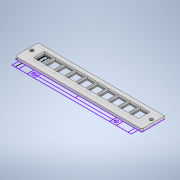
# Autodesk Inventor part: led strip face plate w label addon
Saved by Autodesk Inventor 2022 (Build 260153000, 153)
## iProperties
Created: 2022-04-12
Part Number: led strip face plate w label addon
Material: Generic
Document SubType Name: Modeling
Designer: a-dubs
Density: 1 g/cm^3
Appearance: Default
Author: a-dubs
Autodesk Inventor part; units mm, degrees
ref_plane "YZ Plane" through (0, 0, 0) normal (1, 0, 0) x (0, 1, 0)
ref_plane "XZ Plane" through (0, 0, 0) normal (0, 1, 0) x (-1, 0, 0)
ref_plane "XY Plane" through (0, 0, 0) normal (0, 0, 1) x (1, 0, 0)
sketch "Sketch1" plane through (0, 0, 0) normal (0, 1, 0) x (-1, 0, 0)
  line L0 (0, 0) -> (-9.9, 0)
  line L1 (0, 0) -> (0, -10.3)
  line L2 (0, -10.3) -> (-9.9, -10.3)
  line L3 (-9.9, -10.3) -> (-9.9, 0)
  line L4 (-9.9, -10.3) -> (-9.4, -10.3)
  line L5 (-9.4, -10.3) -> (-9.4, 0)
  line L6 (0, -10.3) -> (-0.5, -10.3)
  line L7 (-0.5, -10.3) -> (-0.5, 0)
  line L8 (-0.5, 0.85) -> (-9.9, 0.85)
  line L9 (-9.9, 0.85) -> (-9.9, 0)
  line L10 (0, 0) -> (0, 0.85)
  line L11 (0, 0.85) -> (-0.5, 0.85)
  line L12 (0, -10.3) -> (0, -11.15)
  line L13 (0, -11.15) -> (-9.9, -11.15)
  line L14 (-9.9, -11.15) -> (-9.9, -10.3)
  line L15 (-9.9, -11.15) -> (-19.8, -11.15)
  line L16 (-19.8, -11.15) -> (-19.8, -10.3)
  line L17 (-19.8, -10.3) -> (-19.8, 0)
  line L18 (-19.3, -10.3) -> (-19.3, 0)
  line L19 (-9.9, -10.3) -> (-19.8, -10.3)
  line L20 (-10.4, -10.3) -> (-10.4, 0)
  line L21 (-9.9, 0) -> (-9.9, -10.3)
  line L22 (-9.9, 0) -> (-9.9, 0.85)
  line L23 (-9.9, 0.85) -> (-10.4, 0.85)
  line L24 (-10.4, 0.85) -> (-19.8, 0.85)
  line L25 (-9.9, 0) -> (-19.8, 0)
  line L26 (-19.8, 0.85) -> (-19.8, 0)
  line L27 (-19.8, -11.15) -> (-29.7, -11.15)
  line L28 (-29.7, -11.15) -> (-29.7, -10.3)
  line L29 (-29.7, -10.3) -> (-29.7, 0)
  line L30 (-29.2, -10.3) -> (-29.2, 0)
  line L31 (-19.8, -10.3) -> (-29.7, -10.3)
  line L32 (-20.3, -10.3) -> (-20.3, 0)
  line L33 (-19.8, 0) -> (-19.8, -10.3)
  line L34 (-19.8, 0) -> (-19.8, 0.85)
  line L35 (-19.8, 0.85) -> (-20.3, 0.85)
  line L36 (-20.3, 0.85) -> (-29.7, 0.85)
  line L37 (-19.8, 0) -> (-29.7, 0)
  line L38 (-29.7, 0.85) -> (-29.7, 0)
  line L39 (-29.7, -11.15) -> (-39.6, -11.15)
  line L40 (-39.6, -11.15) -> (-39.6, -10.3)
  line L41 (-39.6, -10.3) -> (-39.6, 0)
  line L42 (-39.1, -10.3) -> (-39.1, 0)
  line L43 (-29.7, -10.3) -> (-39.6, -10.3)
  line L44 (-30.2, -10.3) -> (-30.2, 0)
  line L45 (-29.7, 0) -> (-29.7, -10.3)
  line L46 (-29.7, 0) -> (-29.7, 0.85)
  line L47 (-29.7, 0.85) -> (-30.2, 0.85)
  line L48 (-30.2, 0.85) -> (-39.6, 0.85)
  line L49 (-29.7, 0) -> (-39.6, 0)
  line L50 (-39.6, 0.85) -> (-39.6, 0)
  line L51 (-39.6, -11.15) -> (-49.5, -11.15)
  line L52 (-49.5, -11.15) -> (-49.5, -10.3)
  line L53 (-49.5, -10.3) -> (-49.5, 0)
  line L54 (-49, -10.3) -> (-49, 0)
  line L55 (-39.6, -10.3) -> (-49.5, -10.3)
  line L56 (-40.1, -10.3) -> (-40.1, 0)
  line L57 (-39.6, 0) -> (-39.6, -10.3)
  line L58 (-39.6, 0) -> (-39.6, 0.85)
  line L59 (-39.6, 0.85) -> (-40.1, 0.85)
  line L60 (-40.1, 0.85) -> (-49.5, 0.85)
  line L61 (-39.6, 0) -> (-49.5, 0)
  line L62 (-49.5, 0.85) -> (-49.5, 0)
  line L63 (-49.5, -11.15) -> (-59.4, -11.15)
  line L64 (-59.4, -11.15) -> (-59.4, -10.3)
  line L65 (-59.4, -10.3) -> (-59.4, 0)
  line L66 (-58.9, -10.3) -> (-58.9, 0)
  line L67 (-49.5, -10.3) -> (-59.4, -10.3)
  line L68 (-50, -10.3) -> (-50, 0)
  line L69 (-49.5, 0) -> (-49.5, -10.3)
  line L70 (-49.5, 0) -> (-49.5, 0.85)
  line L71 (-49.5, 0.85) -> (-50, 0.85)
  line L72 (-50, 0.85) -> (-59.4, 0.85)
  line L73 (-49.5, 0) -> (-59.4, 0)
  line L74 (-59.4, 0.85) -> (-59.4, 0)
  line L75 (-59.4, -11.15) -> (-69.3, -11.15)
  line L76 (-69.3, -11.15) -> (-69.3, -10.3)
  line L77 (-69.3, -10.3) -> (-69.3, 0)
  line L78 (-68.8, -10.3) -> (-68.8, 0)
  line L79 (-59.4, -10.3) -> (-69.3, -10.3)
  line L80 (-59.9, -10.3) -> (-59.9, 0)
  line L81 (-59.4, 0) -> (-59.4, -10.3)
  line L82 (-59.4, 0) -> (-59.4, 0.85)
  line L83 (-59.4, 0.85) -> (-59.9, 0.85)
  line L84 (-59.9, 0.85) -> (-69.3, 0.85)
  line L85 (-59.4, 0) -> (-69.3, 0)
  line L86 (-69.3, 0.85) -> (-69.3, 0)
  line L87 (-69.3, -11.15) -> (-79.2, -11.15)
  line L88 (-79.2, -11.15) -> (-79.2, -10.3)
  line L89 (-79.2, -10.3) -> (-79.2, 0)
  line L90 (-78.7, -10.3) -> (-78.7, 0)
  line L91 (-69.3, -10.3) -> (-79.2, -10.3)
  line L92 (-69.8, -10.3) -> (-69.8, 0)
  line L93 (-69.3, 0) -> (-69.3, -10.3)
  line L94 (-69.3, 0) -> (-69.3, 0.85)
  line L95 (-69.3, 0.85) -> (-69.8, 0.85)
  line L96 (-69.8, 0.85) -> (-79.2, 0.85)
  line L97 (-69.3, 0) -> (-79.2, 0)
  line L98 (-79.2, 0.85) -> (-79.2, 0)
  line L99 (-79.2, -11.15) -> (-89.1, -11.15)
  line L100 (-89.1, -11.15) -> (-89.1, -10.3)
  line L101 (-89.1, -10.3) -> (-89.1, 0)
  line L102 (-88.6, -10.3) -> (-88.6, 0)
  line L103 (-79.2, -10.3) -> (-89.1, -10.3)
  line L104 (-79.7, -10.3) -> (-79.7, 0)
  line L105 (-79.2, 0) -> (-79.2, -10.3)
  line L106 (-79.2, 0) -> (-79.2, 0.85)
  line L107 (-79.2, 0.85) -> (-79.7, 0.85)
  line L108 (-79.7, 0.85) -> (-89.1, 0.85)
  line L109 (-79.2, 0) -> (-89.1, 0)
  line L110 (-89.1, 0.85) -> (-89.1, 0)
  line L111 (-89.1, -11.15) -> (-99, -11.15)
  line L112 (-99, -11.15) -> (-99, -10.3)
  line L113 (-99, -10.3) -> (-99, 0)
  line L114 (-98.5, -10.3) -> (-98.5, 0)
  line L115 (-89.1, -10.3) -> (-99, -10.3)
  line L116 (-89.6, -10.3) -> (-89.6, 0)
  line L117 (-89.1, 0) -> (-89.1, -10.3)
  line L118 (-89.1, 0) -> (-89.1, 0.85)
  line L119 (-89.1, 0.85) -> (-89.6, 0.85)
  line L120 (-89.6, 0.85) -> (-99, 0.85)
  line L121 (-89.1, 0) -> (-99, 0)
  line L122 (-99, 0.85) -> (-99, 0)
  line L123 (0, -11.15) -> (0, 0.85)
  line L124 (0, -11.15) -> (0, -14.15)
  line L125 (0, -14.15) -> (0, -14.15)
  line L126 (-99, 0.85) -> (-102, 0.85)
  line L127 (-102, 0.85) -> (-102, 3.85)
  line L128 (0, -14.15) -> (-102, -14.15)
  line L129 (-102, -14.15) -> (-102, 3.85)
  line L130 (0, 3.89) -> (0, -14.15)
  line L131 (0, -11.15) -> (0, -11.15)
  line L132 (0, 0.85) -> (0, 0.85)
  line L133 (0, -11.15) -> (-2, -11.15)
  line L134 (-2, -11.15) -> (-2, 0.85)
  line L135 (0, -14.15) -> (3.2, -14.15)
  line L136 (3.2, -14.15) -> (3.2, 3.89)
  line L137 (3.2, 3.89) -> (0, 3.89)
  line L138 (0, -11.15) -> (3.2, -11.15)
  line L139 (0, 0.85) -> (3.2, 0.85)
  line L140 (3.2, -14.15) -> (6.2, -14.15)
  line L141 (6.2, 3.89) -> (3.2, 3.89)
  line L142 (0, -14.15) -> (6.2, -14.15)
  line L143 (-49.5, 3.85) -> (-49.5, 0.85)
  line L144 (6.2, 3.89) -> (6.2, 7.09)
  line L145 (6.2, 7.09) -> (6.2, 13.49)
  line L146 (3.2, 3.89) -> (3.2, 13.45)
  line L147 (-102, 3.85) -> (-102, 13.45)
  line L148 (0, 3.89) -> (0, 13.49)
  line L149 (-49.5, 3.85) -> (-87.8335, 3.85)
  line L150 (-49.5, 3.85) -> (-11.1665, 3.89)
  line L151 (-11.1665, 3.89) -> (0, 3.89)
  line L152 (-87.8335, 3.85) -> (-102, 3.85)
  line L153 (-102, -14.15) -> (-105, -14.15)
  line L154 (-105, 13.49) -> (6.2, 13.49)
  line L155 (6.2, 7.09) -> (-105, 7.09)
  line L156 (-49.5, 3.85) -> (-49.5, 7.09)
  line L157 (-49.5, 7.09) -> (-49.5, 10.29)
  line L158 (-49.5, 10.29) -> (-11.1665, 10.29)
  line L159 (-49.5, 10.29) -> (-87.8335, 10.29)
  line L160 (-91.0335, 13.49) -> (-84.6335, 13.49)
  line L161 (-84.6335, 13.49) -> (-84.6335, 7.09)
  line L162 (-84.6335, 7.09) -> (-91.0335, 7.09)
  line L163 (-91.0335, 7.09) -> (-91.0335, 13.49)
  line L164 (-91.0335, 13.49) -> (-84.6335, 7.09) construction
  line L165 (-84.6335, 13.49) -> (-91.0335, 7.09) construction
  line L166 (-14.3665, 13.49) -> (-7.9665, 13.49)
  line L167 (-7.9665, 13.49) -> (-7.9665, 7.09)
  line L168 (-7.9665, 7.09) -> (-14.3665, 7.09)
  line L169 (-14.3665, 7.09) -> (-14.3665, 13.49)
  line L170 (-14.3665, 13.49) -> (-7.9665, 7.09) construction
  line L171 (-7.9665, 13.49) -> (-14.3665, 7.09) construction
  circle A0 centre (-11.1665, 10.29) radius 1.6
  circle A1 centre (-87.8335, 10.29) radius 1.6
  line L172 (6.2, -14.15) -> (9.4, -14.15)
  line L173 (9.4, -14.15) -> (9.4, 3.89)
  line L174 (9.4, 3.89) -> (6.2, 3.89)
  line L175 (9.4, 3.89) -> (9.4, 7.09)
  line L176 (9.4, 7.09) -> (6.2, 7.09)
  line L177 (-105, 7.09) -> (-108.2, 7.09)
  line L178 (-108.2, -14.15) -> (-105, -14.15)
  line L179 (-105, 13.49) -> (-105, 7.09)
  line L180 (-102, -14.15) -> (-108.4, -14.15)
  line L181 (-108.4, -14.15) -> (-108.4, 7.09)
  line L182 (-108.4, 7.09) -> (-108.2, 7.09)
  line L183 (-108.4, -5.13) -> (-105.2, -5.13)
  line L184 (3.2, -11.15) -> (3.2, 0.85)
  line L185 (3.2, -5.15) -> (9.4, -5.15)
  line L186 (3.2, -5.15) -> (9.4, -5.15) construction
  line L187 (9.4, -5.15) -> (6.2, -5.15)
  circle A2 centre (6.2, -5.15) radius 1.6
  circle A3 centre (-105.2, -5.15) radius 1.6
  line L188 (0, 0) -> (-9.9, 0)
  line L189 (-4.95, 0) -> (-4.95, -10.3)
  line L190 (-8.45, -0.95) -> (-1.45, -0.95)
  line L191 (-1.45, -0.95) -> (-1.45, -9.35)
  line L192 (-1.45, -9.35) -> (-8.45, -9.35)
  line L193 (-8.45, -9.35) -> (-8.45, -0.95)
  line L194 (-8.45, -0.95) -> (-1.45, -9.35) construction
  line L195 (-1.45, -0.95) -> (-8.45, -9.35) construction
  line L196 (-9.4, 0) -> (-0.5, 0)
  point P0 (-2, 0)
  point P1 (-2, -10.3)
  point P2 (0, 0.85)
  point P3 (0, 7.09)
  point P4 (3.2, 7.09)
  point P5 (-4.95, -5.15)
  dimension "d0" = 9.9
  dimension "d1" = 10.3
  dimension "d2" = 0.5
  dimension "d3" = 0.5
  dimension "d6" = 0.85
  dimension "d7" = 0.85
  dimension "d10" = 9.9
  dimension "d15" = 3
  dimension "d16" = 0
  dimension "d19" = 3
  dimension "d20" = 2
  dimension "d30" = 3.2
  dimension "d31" = 3
  dimension "d32" = 3
  dimension "d35" = 3.2
  dimension "d36" = 6.4
  dimension "d38" = 38.3335
  dimension "d45" = 3.2
  dimension "d47" = 38.3335
  dimension "d48" = 6.4
  dimension "d49" = 6.4
  dimension "d50" = 3.2
  dimension "d51" = 3.2
  dimension "d53" = 6.4
  dimension "d58" = 3.2
  dimension "d59" = 3.2
  dimension "d60" = 3.2
  dimension "d63" = 7
  dimension "d64" = 8.4
  dimension "d72" = 8.9
  constraints: 394 end point, 68 point on line, 25 perpendicular, 17 horizontal, 10 midpoint, 8 parallel, 7 vertical, 5 collinear, 4 centre point, 4 equal length, 3 coincident, 224 other
  measures "d0" distance of L0.start L0.end
  measures "d1" distance of L0.start L1.end
  measures "d2" distance of L2.end L4.end
  measures "d3" distance of L1.end L6.end
  measures "d6" distance of L0.start L10.end
  measures "d7" distance of L1.end L12.end
  measures "d10" distance of L12.end L15.start
  measures "d15" distance of L12.end L124.end
  measures "d16" distance of L124.end L125.end
  measures "d19" distance of L120.end L126.end
  measures "d20" distance of L12.end L133.end
  measures "d30" distance of L125.end L135.end
  measures "d31" distance of L126.end L127.end
  measures "d32" distance of L135.end L140.end
  measures "d35" distance of L141.start L144.end
  measures "d36" distance of L144.end L145.end
  measures "d38" distance of L143.start L149.end
  measures "d45" distance of L156.end L157.end
  measures "d47" distance of L157.end L158.end
  measures "d48" distance of L161.end L162.end
  measures "d49" distance of L167.end L168.end
  measures "d50" diameter of A0
  measures "d51" distance of L140.end L172.end
  measures "d53" distance of L128.end L180.end
  measures "d58" distance of L186.end L187.end
  measures "d59" diameter of A2
  measures "d60" diameter of A3
  measures "d63" distance of L191.end L192.end
  measures "d64" distance of L190.end L191.end
  measures "d72" distance of L5.end L7.end
extrude "Extrusion6" add sketch "Sketch1" along normal blind 2.4 contours L1 L2 L7 L0 | L10 L139 L136 L138 L12 L1 | L0 L134 L8 L11 L10 | L7 L2 L134 L192 L191 L190 L0 | L12 L13 L134 L2 | L11 L8 L23 L24 L35 L36 L47 L48 L59 L60 L143 L150 L151 L130 | L130 L137 L136 L139 | L134 L190 L189 L0 | L0 L9 L8 L134 | L124 L128 L129 L126 L122 L113 L112 L111 L99 L87 L75 L63 L51 L39 L27 L15 L13 | L138 L136 L135 L124 | L148 L155 L146 L137 | L151 L150 L156 L155 L148 | L136 L141 L174 L173 L185 A2 | L189 L190 L193 L192 L2 L5 L0 | L190 L191 L192 L134 | L134 L192 L189 L190 | L134 L13 L14 L2 | L2 L189 L192 L134 | L136 L185 A2 L173 L172 L140 | L146 L155 L144 L141 | L5 L2 L3 L0 | L189 L192 L193 L190 | L9 L25 L26 L24 L23 | L15 L16 L19 L14 | L153 L178 L180 L181 L182 L177 L155 L147 L127 L129 | L144 L176 L175 L174 | L143 L71 L72 L83 L84 L95 L96 L107 L108 L119 L120 L126 L127 L152 L149 | L149 L152 L147 L155 L156 | L3 L19 L20 L25 | L27 L28 L31 L16 | L60 L59 L50 L61 L62 | L62 L73 L74 L72 L71 | L20 L19 L18 L25 | L26 L37 L38 L36 L35 | L31 L32 L37 L17 | L17 L25 L18 L19 | L39 L40 L43 L28 | L120 L119 L110 L121 L122 | L61 L54 L55 L53 | L53 L67 L68 L73 | L31 L30 L37 L32 | L43 L44 L49 L29 | L29 L37 L30 L31 | L51 L52 L55 L40 | L121 L114 L115 L113 | L48 L47 L38 L49 L50 | L52 L63 L64 L67 | L61 L56 L55 L54 | L68 L67 L66 L73 | L74 L85 L86 L84 L83 | L43 L42 L49 L44 | L55 L56 L61 L41 | L41 L49 L42 L43 | L108 L107 L98 L109 L110 | L115 L100 L111 L112 | L121 L116 L115 L114 | L66 L67 L65 L73 | L65 L79 L80 L85 | L75 L76 L79 L64 | L109 L102 L103 L101 | L101 L115 L116 L121 | L80 L79 L78 L85 | L86 L97 L98 L96 L95 | L87 L88 L91 L76 | L103 L88 L99 L100 | L109 L104 L103 L102 | L78 L79 L77 L85 | L77 L91 L92 L97 | L97 L90 L91 L89 | L89 L103 L104 L109 | L92 L91 L90 L97
extrude "Extrusion7" cut sketch "Sketch1" along normal through all contours L190 L191 L192 L134 | L134 L192 L189 L190 | L189 L192 L193 L190
chamfer "Chamfer2" distance 1 angle 45 4 edges at (4.95, 2.4, -9.35) (1.45, 2.4, -5.15) (8.45, 2.4, -5.15) (4.95, 2.4, -0.95)
pattern_linear "Rectangular Pattern2" count 10 spacing 9.9 along (1, 0, 0) of "Extrusion7", "Chamfer2"
fillet "Fillet1" radius 2 2 edges at (108.4, 1.2, 7.09) (-9.4, 1.2, 7.09)
body "Solid3"
